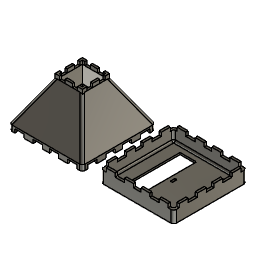
foot_v3 (Autodesk Fusion 360 design; units mm, degrees)
part number: 2025-04-30-06-45-22-033
part number: 2025-04-30-06-45-59-440
part number: 2025-04-30-06-58-08-671
Autodesk Fusion 360 part; units mm, degrees
note: some values were not read from the file. Set by a fixed rule: which sketch regions a step uses.
sketch "Sketch1" plane through (0, 0, 0) normal (0, 0, 1) x (1, 0, 0) in component "bottom_plate"
  line L0 (40, 40) -> (-40, 40)
  line L1 (-40, 40) -> (-40, -40)
  line L2 (-40, -40) -> (40, -40)
  line L3 (40, -40) -> (40, 40)
  line L4 (40, 40) -> (-40, -40) construction
  line L5 (-40, 40) -> (40, -40) construction
  dimension "d1" = 80
  dimension "d2" = 80
  constraint horizontal L0
  constraint perpendicular L0 L1
  constraint parallel L0 L2
  constraint parallel L1 L3
  constraint coincident L4 origin
  constraint coincident L5 origin
  measures "d1" distance of L1.end L2.end
  measures "d2" distance of L0.end L1.end
extrude "Extrude1" add sketch "Sketch1" along normal blind 2 makes body 1 in component "bottom_plate"
sketch "Sketch2" plane through (0, 0, 2) normal (0, 0, 1) x (-1, 0, 0) in component "bottom_plate"
  line L0 (-40, 40) -> (-40, -40)
  line L1 (-40, -40) -> (40, -40)
  line L2 (40, -40) -> (40, 40)
  line L3 (40, 40) -> (-40, 40)
  line L4 (1.1, 2.6) -> (-1.1, 2.6)
  line L5 (-1.1, 2.6) -> (-1.1, -2.6)
  line L6 (-1.1, -2.6) -> (1.1, -2.6)
  line L7 (1.1, -2.6) -> (1.1, 2.6)
  line L8 (1.1, 2.6) -> (-1.1, -2.6) construction
  line L9 (-1.1, 2.6) -> (1.1, -2.6) construction
  dimension "d5" = 2.2
  dimension "d6" = 5.2
  constraint horizontal L4
  constraint perpendicular L4 L5
  constraint parallel L4 L6
  constraint parallel L5 L7
  constraint coincident L8 origin
  constraint coincident L9 origin
  measures "d5" distance of L5.end L6.end
  measures "d6" distance of L4.end L5.end
extrude "Extrude2" cut sketch "Sketch2" against normal blind 2 contours L4 L5 L6 L7 bodies 1 in component "bottom_plate"
sketch "Sketch3" plane through (0, 0, 2) normal (0, 0, 1) x (-1, 0, 0) in component "bottom_plate"
  line L0 (-1.1, 2.6) -> (1.1, 2.6)
  line L1 (1.1, 2.6) -> (1.1, -2.6)
  line L2 (1.1, -2.6) -> (-1.1, -2.6)
  line L3 (-1.1, -2.6) -> (-1.1, 2.6)
  line L4 (-40, 40) -> (-40, -40)
  line L5 (-40, -40) -> (40, -40)
  line L6 (40, -40) -> (40, 40)
  line L7 (40, 40) -> (-40, 40)
  line L8 (40, 0) -> (23, 0) construction
  line L9 (40, -40) -> (23, -40) construction
  line L10 (23, -40) -> (23, -30) construction
  line L11 (23, 0) -> (14, 0) construction
  line L12 (23, -30) -> (5, -30)
  line L13 (5, -30) -> (5, 30)
  line L14 (5, 30) -> (23, 30)
  line L15 (23, 30) -> (23, -30)
  line L16 (23, -30) -> (5, 30) construction
  line L17 (5, -30) -> (23, 30) construction
  point P0 (14, 0)
  dimension "d9" = 17
  dimension "d10" = 17
  dimension "d11" = 10
  dimension "d12" = 9
  constraint midpoint L6 L8.start
  constraint perpendicular L4 L8
  constraint coincident L5.end L6.start
  constraint coincident L5 L9.end
  constraint perpendicular L5 L10
  constraint parallel L8 L11
  constraint horizontal L12
  constraint perpendicular L12 L13
  constraint parallel L12 L14
  constraint parallel L13 L15
  constraint coincident L16 P0
  constraint coincident L17 P0
  constraint coincident P0 L11.end
  measures "d9" distance of L8.start L8.end
  measures "d10" distance of L5.end L9.end
  measures "d11" distance of L9.end L10.end
  measures "d12" distance of L8.end P0
extrude "Extrude3" cut sketch "Sketch3" against normal blind 2 contours L12 L13 L14 L15 bodies 1 in component "bottom_plate"
sketch "Sketch1 (2)" plane through (0, 0, 0) normal (0, 0, 1) x (1, 0, 0) in component "top"
  line L0 (40, -40) -> (-40, -40)
  line L1 (-40, -40) -> (-40, 40)
  line L2 (-40, 40) -> (40, 40)
  line L3 (40, 40) -> (40, -40)
  constraint horizontal L0
  constraint vertical L1
  constraint horizontal L2
  constraint vertical L3
extrude "Extrude1'" add sketch "Sketch1 (2)" along normal blind 43.5 separate body makes body 2 in component "top"
ref_plane "WorkPlane1" through (0, 40, 0) normal (0, 1, 0) x (0, 0, 1) in component "top"
ref_plane "WorkPlane2" through (40, 0, 0) normal (1, 0, 0) x (0, 1, 0) in component "top"
sketch "Sketch2 (2)" plane through (0, 40, 0) normal (0, 1, 0) x (1, 0, 0) in component "top"
  line L0 (0, -43.5) -> (-15, -43.5) construction
  line L1 (-15, -43.5) -> (0, -43.5) construction
  line L2 (0, -43.5) -> (15, -43.5) construction
  line L3 (15, -43.5) -> (40, 0)
  line L4 (40, 0) -> (40, -43.5)
  line L5 (40, -43.5) -> (15, -43.5)
  line L6 (-15, -43.5) -> (-40, 0)
  line L7 (-40, 0) -> (-40, -43.5)
  line L8 (-40, -43.5) -> (-15, -43.5)
  dimension "d41" = 15
  dimension "d42" = 15
  constraint horizontal L0
  constraint parallel L0 L2
  constraint perpendicular L2 L4
  constraint perpendicular L4 L5
  constraint perpendicular L1 L7
  constraint perpendicular L7 L8
  measures "d41" distance of L0.start L0.end
  measures "d42" distance of L0.start L2.end
extrude "Extrude2'" cut sketch "Sketch2 (2)" against normal blind 80 bodies 2 in component "top"
sketch "Sketch3 (2)" plane through (40, 0, 0) normal (1, 0, 0) x (0, 1, 0) in component "top"
  line L0 (0, 43.5) -> (-15, 43.5) construction
  line L1 (0, 43.5) -> (15, 43.5) construction
  line L2 (15, 43.5) -> (40, 0)
  line L3 (40, 0) -> (40, 43.5)
  line L4 (40, 43.5) -> (15, 43.5)
  line L5 (-15, 43.5) -> (-40, 43.5)
  line L6 (-40, 43.5) -> (-40, 0)
  line L7 (-40, 0) -> (-15, 43.5)
  dimension "d45" = 15
  dimension "d46" = 15
  constraint horizontal L0
  constraint parallel L0 L1
  constraint perpendicular L1 L3
  constraint perpendicular L3 L4
  constraint parallel L0 L5
  constraint perpendicular L5 L6
  measures "d45" distance of L0.start L0.end
  measures "d46" distance of L0.start L1.end
extrude "Extrude3'" cut sketch "Sketch3 (2)" against normal blind 80 bodies 2 in component "top"
shell "Shell1" thickness 2 removed faces 2 at (13.3333, -13.3333, 0) at (5, -5, 43.5) on bodies 2 in component "top"
sketch "Sketch4" plane through (0, 0, 43.5) normal (0, 0, 1) x (-1, 0, 0) in component "top"
  line L0 (-12.6932, 12.6932) -> (12.6932, 12.6932)
  line L1 (12.6932, 12.6932) -> (12.6932, -12.6932)
  line L2 (12.6932, -12.6932) -> (-12.6932, -12.6932)
  line L3 (-12.6932, -12.6932) -> (-12.6932, 12.6932)
  line L4 (-15, -15) -> (15, -15)
  line L5 (15, -15) -> (15, 15)
  line L6 (15, 15) -> (-15, 15)
  line L7 (-15, 15) -> (-15, -15)
  line L8 (-15, 15) -> (15, 15) construction
  line L9 (15, 15) -> (15, 12.693) construction
  line L10 (15, 12.693) -> (-15, 12.693) construction
  line L11 (-15, 12.693) -> (-15, 15) construction
  line L12 (-15, 15) -> (-12.6932, 15) construction
  line L13 (-12.6932, 15) -> (-12.6932, -15) construction
  line L14 (-12.6932, -15) -> (-15, -15) construction
  line L15 (-15, -15) -> (-15, 15) construction
  line L16 (-15, 15) -> (-10, 15)
  line L17 (-10, 15) -> (-10, 12.693)
  line L18 (-10, 12.693) -> (-15, 12.693)
  line L19 (-15, 12.693) -> (-15, 15)
  line L20 (-10, 15) -> (-4, 15) construction
  line L21 (-4, 15) -> (-4, 12.6932) construction
  line L22 (-4, 12.6932) -> (-10, 12.6932) construction
  line L23 (-10, 12.6932) -> (-10, 15) construction
  line L24 (-4, 15) -> (0, 15)
  line L25 (0, 15) -> (0, 12.693)
  line L26 (0, 12.693) -> (-4, 12.693)
  line L27 (-4, 12.693) -> (-4, 15)
  line L28 (-15, 15) -> (-12.6932, 15)
  line L29 (-12.6932, 15) -> (-12.6932, 10)
  line L30 (-12.6932, 10) -> (-15, 10)
  line L31 (-15, 10) -> (-15, 15)
  line L32 (-15, 10) -> (-12.6932, 10) construction
  line L33 (-12.6932, 10) -> (-12.6932, 4) construction
  line L34 (-12.6932, 4) -> (-15, 4) construction
  line L35 (-15, 4) -> (-15, 10) construction
  line L36 (-15, 4) -> (-12.6932, 4)
  line L37 (-12.6932, 4) -> (-12.6932, 0)
  line L38 (-12.6932, 0) -> (-15, 0)
  line L39 (-15, 0) -> (-15, 4)
  dimension "d50" = 30
  dimension "d51" = 2.307
  dimension "d52" = 30
  dimension "d53" = 5
  dimension "d54" = 6
  dimension "d55" = 5
  dimension "d56" = 6
  constraint horizontal L8
  constraint vertical L9
  constraint horizontal L10
  constraint vertical L11
  constraint coincident L6.end L7.start
  constraint horizontal L12
  constraint vertical L13
  constraint horizontal L14
  constraint vertical L15
  constraint horizontal L16
  constraint vertical L17
  constraint horizontal L18
  constraint vertical L19
  constraint coincident L10 L17.end
  constraint horizontal L20
  constraint vertical L21
  constraint horizontal L22
  constraint vertical L23
  constraint coincident L0 L21.end
  constraint horizontal L24
  constraint vertical L25
  constraint horizontal L26
  constraint vertical L27
  constraint midpoint L10 L25.end
  constraint horizontal L28
  constraint vertical L29
  constraint horizontal L30
  constraint vertical L31
  constraint horizontal L32
  constraint vertical L33
  constraint horizontal L34
  constraint vertical L35
  constraint horizontal L36
  constraint vertical L37
  constraint horizontal L38
  constraint vertical L39
  constraint midpoint L13 L37.end
  measures "d50" distance of L6.end L5.end
  measures "d51" distance of L6.end L10.end
  measures "d52" distance of L6.end L4.start
  measures "d53" distance of L6.end L16.end
  measures "d54" distance of L16.end L20.end
  measures "d55" distance of L6.end L30.end
  measures "d56" distance of L30.end L34.end
extrude "Extrude4" add sketch "Sketch4" along normal blind 4 contours L0 L6 L16 L17 L18 L29 | L3 L7 L18 L29 L30 L31 | L6 L7 L16 L18 L19 L28 L29 L31 | L0 L6 L24 L25 L26 L27 | L3 L7 L36 L37 L38 L39 bodies 2 in component "top"
mirror "Mirror1" about plane through (0, 0, 0) normal (1, 0, 0) of "Extrude4" in component "top"
mirror "Mirror2" about plane through (0, 0, 0) normal (0, 1, 0) of "Extrude4", "Mirror1" in component "top"
sketch "Sketch6" plane through (0, 0, 2) normal (0, 0, 1) x (-1, 0, 0) in component "bottom_plate"
  line L0 (5, -30) -> (5, 30)
  line L1 (5, 30) -> (23, 30)
  line L2 (23, 30) -> (23, -30)
  line L3 (23, -30) -> (5, -30)
  line L4 (-1.1, 2.6) -> (1.1, 2.6)
  line L5 (1.1, 2.6) -> (1.1, -2.6)
  line L6 (1.1, -2.6) -> (-1.1, -2.6)
  line L7 (-1.1, -2.6) -> (-1.1, 2.6)
  line L8 (-40, 40) -> (-40, -40)
  line L9 (-40, -40) -> (40, -40)
  line L10 (40, -40) -> (40, 40)
  line L11 (40, 40) -> (-40, 40)
  line L12 (-40, 40) -> (40, 40)
  line L13 (40, 40) -> (40, 37.5)
  line L14 (40, 37.5) -> (-40, 37.5)
  line L15 (-40, 37.5) -> (-40, 40)
  line L16 (-40, 40) -> (-37.5, 40)
  line L17 (-37.5, 40) -> (-37.5, -40)
  line L18 (-37.5, -40) -> (-40, -40)
  line L19 (-40, -40) -> (-40, 40)
  line L20 (-40, -40) -> (40, -40)
  line L21 (40, -40) -> (40, -37.5)
  line L22 (40, -37.5) -> (-40, -37.5)
  line L23 (-40, -37.5) -> (-40, -40)
  line L24 (40, -40) -> (37.5, -40)
  line L25 (37.5, -40) -> (37.5, 40)
  line L26 (37.5, 40) -> (40, 40)
  line L27 (40, 40) -> (40, -40)
  dimension "d93" = 2.5
  dimension "d94" = 2.5
  dimension "d95" = 80
  dimension "d96" = 2.5
  dimension "d97" = 2.5
  dimension "d98" = 80
  constraint horizontal L12
  constraint vertical L13
  constraint horizontal L14
  constraint vertical L15
  constraint coincident L10 L13.end
  constraint coincident L8.start L11.end
  constraint horizontal L16
  constraint vertical L17
  constraint horizontal L18
  constraint vertical L19
  constraint horizontal L20
  constraint vertical L21
  constraint horizontal L22
  constraint vertical L23
  constraint coincident L8.end L9.start
  constraint horizontal L24
  constraint vertical L25
  constraint horizontal L26
  constraint vertical L27
  constraint coincident L9.end L10.start
  measures "d93" distance of L8.start L14.end
  measures "d94" distance of L8.start L16.end
  measures "d95" distance of L8.start L8.end
  measures "d96" distance of L8.end L22.end
  measures "d97" distance of L9.end L24.end
  measures "d98" distance of L9.end L10.end
extrude "Extrude6" add sketch "Sketch6" along normal blind 15 contours L8 L11 L12 L14 L15 L16 L17 L19 | L8 L14 L17 L19 L22 | L11 L12 L14 L17 L25 | L8 L9 L17 L18 L19 L20 L22 L23 | L10 L11 L12 L13 L14 L25 L26 L27 | L9 L17 L20 L22 L25 | L10 L14 L22 L25 L27 | L9 L10 L20 L21 L22 L24 L25 L27 bodies 1 in component "bottom_plate"
sketch "Sketch7" plane through (0, 0, 17) normal (0, 0, 1) x (-1, 0, 0) in component "bottom_plate"
  line L0 (-37.5, 37.5) -> (37.5, 37.5)
  line L1 (37.5, 37.5) -> (37.5, -37.5)
  line L2 (37.5, -37.5) -> (-37.5, -37.5)
  line L3 (-37.5, -37.5) -> (-37.5, 37.5)
  line L4 (-40, 40) -> (-40, -40)
  line L5 (-40, -40) -> (40, -40)
  line L6 (40, -40) -> (40, 40)
  line L7 (40, 40) -> (-40, 40)
  line L8 (-40, 40) -> (40, 40) construction
  line L9 (40, 40) -> (40, 37.5) construction
  line L10 (40, 37.5) -> (-40, 37.5) construction
  line L11 (-40, 37.5) -> (-40, 40) construction
  line L12 (-40, 40) -> (-37.5, 40) construction
  line L13 (-37.5, 40) -> (-37.5, -40) construction
  line L14 (-37.5, -40) -> (-40, -40) construction
  line L15 (-40, -40) -> (-40, 40) construction
  line L16 (-40, 40) -> (-33.9, 40)
  line L17 (-33.9, 40) -> (-33.9, 37.5)
  line L18 (-33.9, 37.5) -> (-40, 37.5)
  line L19 (-40, 37.5) -> (-40, 40)
  line L20 (-40, 40) -> (-37.5, 40)
  line L21 (-37.5, 40) -> (-37.5, 33.9)
  line L22 (-37.5, 33.9) -> (-40, 33.9)
  line L23 (-40, 33.9) -> (-40, 40)
  line L24 (-33.9, 40) -> (-24.1, 40) construction
  line L25 (-24.1, 40) -> (-24.1, 37.5) construction
  line L26 (-24.1, 37.5) -> (-33.9, 37.5) construction
  line L27 (-33.9, 37.5) -> (-33.9, 40) construction
  line L28 (-24.1, 40) -> (-13.9, 40)
  line L29 (-13.9, 40) -> (-13.9, 37.5)
  line L30 (-13.9, 37.5) -> (-24.1, 37.5)
  line L31 (-24.1, 37.5) -> (-24.1, 40)
  line L32 (-13.9, 40) -> (-4.1, 40) construction
  line L33 (-4.1, 40) -> (-4.1, 37.5) construction
  line L34 (-4.1, 37.5) -> (-13.9, 37.5) construction
  line L35 (-13.9, 37.5) -> (-13.9, 40) construction
  line L36 (-4.1, 40) -> (0, 40)
  line L37 (0, 40) -> (0, 37.5)
  line L38 (0, 37.5) -> (-4.1, 37.5)
  line L39 (-4.1, 37.5) -> (-4.1, 40)
  line L40 (-40, 33.9) -> (-37.5, 33.9) construction
  line L41 (-37.5, 33.9) -> (-37.5, 24.1) construction
  line L42 (-37.5, 24.1) -> (-40, 24.1) construction
  line L43 (-40, 24.1) -> (-40, 33.9) construction
  line L44 (-40, 24.1) -> (-37.5, 24.1)
  line L45 (-37.5, 24.1) -> (-37.5, 13.9)
  line L46 (-37.5, 13.9) -> (-40, 13.9)
  line L47 (-40, 13.9) -> (-40, 24.1)
  line L48 (-40, 13.9) -> (-37.5, 13.9) construction
  line L49 (-37.5, 13.9) -> (-37.5, 4.1) construction
  line L50 (-37.5, 4.1) -> (-40, 4.1) construction
  line L51 (-40, 4.1) -> (-40, 13.9) construction
  line L52 (-40, 4.1) -> (-37.5, 4.1)
  line L53 (-37.5, 4.1) -> (-37.5, 0)
  line L54 (-37.5, 0) -> (-40, 0)
  line L55 (-40, 0) -> (-40, 4.1)
  dimension "d101" = 6.1
  dimension "d102" = 6.1
  dimension "d103" = 9.8
  dimension "d104" = 10.2
  dimension "d105" = 9.8
  dimension "d106" = 9.8
  dimension "d107" = 10.2
  dimension "d108" = 9.8
  constraint horizontal L8
  constraint vertical L9
  constraint horizontal L10
  constraint vertical L11
  constraint coincident L6 L9.end
  constraint coincident L4.start L7.end
  constraint horizontal L12
  constraint vertical L13
  constraint horizontal L14
  constraint vertical L15
  constraint coincident L5 L13.end
  constraint horizontal L16
  constraint vertical L17
  constraint horizontal L18
  constraint vertical L19
  constraint coincident L0 L17.end
  constraint coincident L10 L17.end
  constraint horizontal L20
  constraint vertical L21
  constraint horizontal L22
  constraint vertical L23
  constraint coincident L3 L21.end
  constraint coincident L13 L21.end
  constraint horizontal L24
  constraint vertical L25
  constraint horizontal L26
  constraint vertical L27
  constraint coincident L0 L25.end
  constraint horizontal L28
  constraint vertical L29
  constraint horizontal L30
  constraint vertical L31
  constraint coincident L0 L29.end
  constraint horizontal L32
  constraint vertical L33
  constraint horizontal L34
  constraint vertical L35
  constraint coincident L10 L33.end
  constraint horizontal L36
  constraint vertical L37
  constraint horizontal L38
  constraint vertical L39
  constraint midpoint L10 L37.end
  constraint horizontal L40
  constraint vertical L41
  constraint horizontal L42
  constraint vertical L43
  constraint coincident L13 L41.end
  constraint horizontal L44
  constraint vertical L45
  constraint horizontal L46
  constraint vertical L47
  constraint coincident L3 L45.end
  constraint horizontal L48
  constraint vertical L49
  constraint horizontal L50
  constraint vertical L51
  constraint coincident L13 L49.end
  constraint horizontal L52
  constraint vertical L53
  constraint horizontal L54
  constraint vertical L55
  constraint midpoint L13 L53.end
  measures "d101" distance of L4.start L16.end
  measures "d102" distance of L4.start L22.end
  measures "d103" distance of L16.end L24.end
  measures "d104" distance of L24.end L28.end
  measures "d105" distance of L28.end L32.end
  measures "d106" distance of L22.end L42.end
  measures "d107" distance of L42.end L46.end
  measures "d108" distance of L46.end L50.end
extrude "Extrude7" cut sketch "Sketch7" against normal blind 4 contours L0 L7 L16 L17 L18 L21 | L3 L4 L18 L21 L22 L23 | L4 L7 L16 L18 L19 L20 L21 L23 | L0 L7 L28 L29 L30 L31 | L3 L4 L44 L45 L46 L47 | L0 L7 L36 L37 L38 L39 | L3 L4 L52 L53 L54 L55 bodies 1 in component "bottom_plate"
mirror "Mirror3" about plane through (0, 0, 0) normal (1, 0, 0) of "Extrude7" in component "bottom_plate"
mirror "Mirror4" about plane through (0, 0, 0) normal (0, 1, 0) of "Extrude7", "Mirror3" in component "bottom_plate"
fillet "Fillet5" radius 3 4 edges at (40, 40, 6.5) (-40, 40, 6.5) (-40, -40, 6.5) (40, -40, 6.5) on bodies 1 in component "bottom_plate"
fillet "Fillet6" radius 2 4 edges at (-37.5, -37.5, 7.5) (37.5, -37.5, 7.5) (-37.5, 37.5, 7.5) (37.5, 37.5, 7.5) on bodies 1 in component "bottom_plate"
fillet "Fillet7" radius 2 8 edges at (-37.5, 0, 2) (-36.9142, -36.9142, 2) (0, -37.5, 2) (36.9142, -36.9142, 2) (37.5, 0, 2) (36.9142, 36.9142, 2) (0, 37.5, 2) (-36.9142, 36.9142, 2) on bodies 1 in component "bottom_plate"
sketch "Sketch6 (2)" plane through (0, 0, 0) normal (0, 0, -1) x (1, 0, 0) in component "top"
  line L0 (-37.6932, 37.6932) -> (37.6932, 37.6932)
  line L1 (37.6932, 37.6932) -> (37.6932, -37.6932)
  line L2 (37.6932, -37.6932) -> (-37.6932, -37.6932)
  line L3 (-37.6932, -37.6932) -> (-37.6932, 37.6932)
  line L4 (-40, -40) -> (40, -40)
  line L5 (40, -40) -> (40, 40)
  line L6 (40, 40) -> (-40, 40)
  line L7 (-40, 40) -> (-40, -40)
  line L8 (-40, 40) -> (40, 40)
  line L9 (40, 40) -> (40, 37.693)
  line L10 (40, 37.693) -> (-40, 37.693)
  line L11 (-40, 37.693) -> (-40, 40)
  line L12 (-40, 40) -> (-37.693, 40)
  line L13 (-37.693, 40) -> (-37.693, -40)
  line L14 (-37.693, -40) -> (-40, -40)
  line L15 (-40, -40) -> (-40, 40)
  line L16 (-40, -40) -> (40, -40)
  line L17 (40, -40) -> (40, -37.693)
  line L18 (40, -37.693) -> (-40, -37.693)
  line L19 (-40, -37.693) -> (-40, -40)
  line L20 (40, -40) -> (37.693, -40)
  line L21 (37.693, -40) -> (37.693, 40)
  line L22 (37.693, 40) -> (40, 40)
  line L23 (40, 40) -> (40, -40)
  dimension "d121" = 80
  dimension "d122" = 2.307
  dimension "d123" = 2.307
  dimension "d124" = 80
  dimension "d125" = 80
  dimension "d126" = 2.307
  dimension "d127" = 2.307
  dimension "d128" = 80
  constraint horizontal L8
  constraint vertical L9
  constraint horizontal L10
  constraint vertical L11
  constraint coincident L6.end L7.start
  constraint horizontal L12
  constraint vertical L13
  constraint horizontal L14
  constraint vertical L15
  constraint horizontal L16
  constraint vertical L17
  constraint horizontal L18
  constraint vertical L19
  constraint coincident L4.start L7.end
  constraint horizontal L20
  constraint vertical L21
  constraint horizontal L22
  constraint vertical L23
  constraint coincident L4.end L5.start
  measures "d121" distance of L6.end L5.end
  measures "d122" distance of L6.end L10.end
  measures "d123" distance of L6.end L12.end
  measures "d124" distance of L6.end L4.start
  measures "d125" distance of L4.start L4.end
  measures "d126" distance of L4.start L18.end
  measures "d127" distance of L4.end L20.end
  measures "d128" distance of L4.end L5.end
extrude "Extrude6'" add sketch "Sketch6 (2)" along normal blind 2 contours L0 L6 L8 L10 L13 L21 | L3 L7 L10 L13 L15 L18 | L6 L7 L8 L10 L11 L12 L13 L15 | L1 L5 L10 L18 L21 L23 | L5 L6 L8 L9 L10 L21 L22 L23 | L2 L4 L13 L16 L18 L21 | L4 L7 L13 L14 L15 L16 L18 L19 | L4 L5 L16 L17 L18 L20 L21 L23 bodies 2 in component "top"
sketch "Sketch7 (2)" plane through (0, 0, -2) normal (0, 0, -1) x (1, 0, 0) in component "top"
  line L0 (37.6932, -37.6932) -> (-37.6932, -37.6932)
  line L1 (-37.6932, -37.6932) -> (-37.6932, 37.6932)
  line L2 (-37.6932, 37.6932) -> (37.6932, 37.6932)
  line L3 (37.6932, 37.6932) -> (37.6932, -37.6932)
  line L4 (-40, 40) -> (-40, -40)
  line L5 (-40, -40) -> (40, -40)
  line L6 (40, -40) -> (40, 40)
  line L7 (40, 40) -> (-40, 40)
  line L8 (-40, 40) -> (40, 40) construction
  line L9 (40, 40) -> (40, 37.6932) construction
  line L10 (40, 37.6932) -> (-40, 37.6932) construction
  line L11 (-40, 37.6932) -> (-40, 40) construction
  line L12 (-40, 40) -> (-37.6932, 40) construction
  line L13 (-37.6932, 40) -> (-37.6932, -40) construction
  line L14 (-37.6932, -40) -> (-40, -40) construction
  line L15 (-40, -40) -> (-40, 40) construction
  line L16 (-40, 40) -> (-34, 40)
  line L17 (-34, 40) -> (-34, 37.6932)
  line L18 (-34, 37.6932) -> (-40, 37.6932)
  line L19 (-40, 37.6932) -> (-40, 40)
  line L20 (-34, 40) -> (-24, 40) construction
  line L21 (-24, 40) -> (-24, 37.6932) construction
  line L22 (-24, 37.6932) -> (-34, 37.6932) construction
  line L23 (-34, 37.6932) -> (-34, 40) construction
  line L24 (-24, 40) -> (-14, 40)
  line L25 (-14, 40) -> (-14, 37.6932)
  line L26 (-14, 37.6932) -> (-24, 37.6932)
  line L27 (-24, 37.6932) -> (-24, 40)
  line L28 (-14, 40) -> (-4, 40) construction
  line L29 (-4, 40) -> (-4, 37.6932) construction
  line L30 (-4, 37.6932) -> (-14, 37.6932) construction
  line L31 (-14, 37.6932) -> (-14, 40) construction
  line L32 (-4, 40) -> (0, 40)
  line L33 (0, 40) -> (0, 37.6932)
  line L34 (0, 37.6932) -> (-4, 37.6932)
  line L35 (-4, 37.6932) -> (-4, 40)
  line L36 (-40, 40) -> (-37.6932, 40)
  line L37 (-37.6932, 40) -> (-37.6932, 34)
  line L38 (-37.6932, 34) -> (-40, 34)
  line L39 (-40, 34) -> (-40, 40)
  line L40 (-40, 34) -> (-37.6932, 34) construction
  line L41 (-37.6932, 34) -> (-37.6932, 24) construction
  line L42 (-37.6932, 24) -> (-40, 24) construction
  line L43 (-40, 24) -> (-40, 34) construction
  line L44 (-40, 24) -> (-37.6932, 24)
  line L45 (-37.6932, 24) -> (-37.6932, 14)
  line L46 (-37.6932, 14) -> (-40, 14)
  line L47 (-40, 14) -> (-40, 24)
  line L48 (-40, 14) -> (-37.6932, 14) construction
  line L49 (-37.6932, 14) -> (-37.6932, 4) construction
  line L50 (-37.6932, 4) -> (-40, 4) construction
  line L51 (-40, 4) -> (-40, 14) construction
  line L52 (-40, 4) -> (-37.6932, 4)
  line L53 (-37.6932, 4) -> (-37.6932, 0)
  line L54 (-37.6932, 0) -> (-40, 0)
  line L55 (-40, 0) -> (-40, 4)
  dimension "d131" = 6
  dimension "d132" = 10
  dimension "d133" = 10
  dimension "d134" = 10
  dimension "d135" = 6
  dimension "d136" = 10
  dimension "d137" = 10
  dimension "d138" = 10
  constraint horizontal L8
  constraint vertical L9
  constraint horizontal L10
  constraint vertical L11
  constraint coincident L6 L9.end
  constraint coincident L4.start L7.end
  constraint horizontal L12
  constraint vertical L13
  constraint horizontal L14
  constraint vertical L15
  constraint coincident L5 L13.end
  constraint horizontal L16
  constraint vertical L17
  constraint horizontal L18
  constraint vertical L19
  constraint coincident L10 L17.end
  constraint coincident L2 L17.end
  constraint horizontal L20
  constraint vertical L21
  constraint horizontal L22
  constraint vertical L23
  constraint coincident L2 L21.end
  constraint horizontal L24
  constraint vertical L25
  constraint horizontal L26
  constraint vertical L27
  constraint coincident L10 L25.end
  constraint horizontal L28
  constraint vertical L29
  constraint horizontal L30
  constraint vertical L31
  constraint coincident L10 L29.end
  constraint horizontal L32
  constraint vertical L33
  constraint horizontal L34
  constraint vertical L35
  constraint midpoint L2 L33.end
  constraint horizontal L36
  constraint vertical L37
  constraint horizontal L38
  constraint vertical L39
  constraint coincident L13 L37.end
  constraint coincident L1 L37.end
  constraint horizontal L40
  constraint vertical L41
  constraint horizontal L42
  constraint vertical L43
  constraint coincident L13 L41.end
  constraint horizontal L44
  constraint vertical L45
  constraint horizontal L46
  constraint vertical L47
  constraint coincident L1 L45.end
  constraint horizontal L48
  constraint vertical L49
  constraint horizontal L50
  constraint vertical L51
  constraint coincident L13 L49.end
  constraint horizontal L52
  constraint vertical L53
  constraint horizontal L54
  constraint vertical L55
  constraint midpoint L13 L53.end
  measures "d131" distance of L4.start L16.end
  measures "d132" distance of L16.end L20.end
  measures "d133" distance of L20.end L24.end
  measures "d134" distance of L24.end L28.end
  measures "d135" distance of L4.start L38.end
  measures "d136" distance of L38.end L42.end
  measures "d137" distance of L42.end L46.end
  measures "d138" distance of L46.end L50.end
extrude "Extrude7'" add sketch "Sketch7 (2)" along normal blind 4 contours L1 L4 L52 L53 L54 L55 | L2 L7 L32 L33 L34 L35 | L1 L4 L44 L45 L46 L47 | L2 L7 L24 L25 L26 L27 | L1 L4 L18 L37 L38 L39 | L2 L7 L16 L17 L18 L37 | L4 L7 L16 L18 L19 L36 L37 L39 bodies 2 in component "top"
mirror "Mirror5" about plane through (0, 0, -4) normal (1, 0, 0) of "Extrude7'" in component "top"
mirror "Mirror6" about plane through (0, 0, -4) normal (0, 1, 0) of "Extrude7'", "Mirror5" in component "top"
fillet "Fillet4" radius 3 8 edges at (-27.5, 27.5, 21.75) (27.5, 27.5, 21.75) (27.5, -27.5, 21.75) (-27.5, -27.5, 21.75) (40, -40, -3) (-40, -40, -3) (-40, 40, -3) (40, 40, -3) on bodies 2 in component "top"
component "bottom_plate" placed x (1, 0, 0) y (0, 1, 0) z (0, 0, 1) at (100, 0, 0)
component "top" placed x (1, 0, 0) y (0, 1, 0) z (0, 0, 1) at (0, 0, 4)
